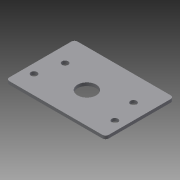
# Autodesk Inventor part: motorMount
Saved by Autodesk Inventor 2013 (Build 170138000, 138)
## iProperties
Created: 2012-12-12
Part Number: motorMount
Material: Generic
Document SubType Name: Modeling
Designer: istvan.burbank
Density: 1 g/cm^3
Author: istvan.burbank
Autodesk Inventor part; units mm, degrees
ref_plane "YZ Plane" through (0, 0, 0) normal (1, 0, 0) x (0, 1, 0)
ref_plane "XZ Plane" through (0, 0, 0) normal (0, 1, 0) x (-1, 0, 0)
ref_plane "XY Plane" through (0, 0, 0) normal (0, 0, 1) x (1, 0, 0)
sketch "Sketch1" plane through (0, 0, 0) normal (0, 1, 0) x (-1, 0, 0)
  line L0 (3.175, 0) -> (98.425, 0)
  line L1 (101.6, 3.175) -> (101.6, 66.675)
  line L2 (98.425, 69.85) -> (3.175, 69.85)
  line L3 (0, 66.675) -> (0, 3.175)
  arc A0 (3.175, 69.85) -> (0, 66.675) centre (3.175, 66.675) ccw
  arc A1 (101.6, 66.675) -> (98.425, 69.85) centre (98.425, 66.675) ccw
  arc A2 (98.425, 0) -> (101.6, 3.175) centre (98.425, 3.175) ccw
  arc A3 (0, 3.175) -> (3.175, 0) centre (3.175, 3.175) ccw
  point P0 (0, 0)
  point P1 (101.6, 69.85)
  point P2 (101.6, 0)
  point P3 (0, 69.85)
  dimension "d0" = 101.6
  dimension "d1" = 69.85
  dimension "d13" = 3.175
  constraints: 8 end point, 8 point on circle, 8 point on line, 8 tangent, 4 centre point, 3 equal radius, 2 parallel, 1 horizontal, 1 perpendicular
  measures "d0" distance of point (0, 69.85) point (101.6, 69.85)
  measures "d1" distance of point (101.6, 69.85) point (101.6, 0)
  measures "d13" radius of A0
extrude "Extrusion1" add sketch "Sketch1" along normal blind 3.175
sketch "Sketch2" plane through (0, 3.175, 0) normal (0, 1, 0) x (1, 0, 0)
  line L0 (-3.175, 0) -> (-98.425, 0) projected
  line L1 (-101.6, -3.175) -> (-101.6, -66.675) projected
  line L2 (0, -66.675) -> (0, -3.175) projected
  point P0 (0, 0)
  point P1 (-76.2, 0)
  point P2 (-76.2, -76.2)
  point P3 (-50.8, -38.1)
  dimension "d4" = 50.8
  dimension "d5" = 38.1
  dimension "d29" = 50.8
  constraints: 1 other
  measures "d5" distance from line of L0 point (-50.8, -38.1)
  measures "d29" distance from line of L2 point (-50.8, -38.1)
hole "Hole1" at (-50.8, 3.175, 38.1) direction (0, -1, 0) diameter 19.05 end through all
sketch "Sketch3" plane through (0, 3.175, 0) normal (0, 1, 0) x (1, 0, 0)
  line L0 (0, -66.675) -> (0, -3.175) projected
  line L1 (-101.6, -3.175) -> (-101.6, -66.675) projected
  circle A0 centre (-50.8, -38.1) radius 9.525 projected
  point P0 (0, 0)
  point P1 (-85.725, -25.4)
  point P2 (-15.875, -25.4)
  point P3 (-9.525, -50.8)
  point P4 (-92.075, -50.8)
  dimension "d30" = 6.35
  dimension "d33" = 25.4
  dimension "d36" = 9.525
  dimension "d37" = 9.525
  dimension "d38" = 6.35
  dimension "d39" = 12.7
  dimension "d40" = 82.55
  constraints: 2 horizontal alignment
  measures "d30" horizontal distance of point (-9.525, -50.8) point (-15.875, -25.4)
  measures "d33" vertical distance of point (-9.525, -50.8) point (-15.875, -25.4)
  measures "d36" distance from line of L1 point (-92.075, -50.8)
  measures "d37" distance from line of L0 point (-9.525, -50.8)
  measures "d38" horizontal distance of point (-92.075, -50.8) point (-85.725, -25.4)
  measures "d39" vertical distance of point (-9.525, -50.8) A0.centre
  measures "d40" distance of point (-9.525, -50.8) point (-92.075, -50.8)
hole "Hole2" at (-85.725, 3.175, 25.4) at (-15.875, 3.175, 25.4) at (-9.525, 3.175, 50.8) at (-92.075, 3.175, 50.8) direction (0, -1, 0) diameter 6.35 end through all
equation "\"d4\" = d29"
equation "\"d36\" = d37"
equation "\"d38\" = d30"
body "Solid1"
